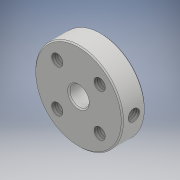
# Autodesk Inventor part: pololu-mounting-hub
Saved by Autodesk Inventor 2018 (Build 220112000, 112)
## iProperties
Created: 2017-11-16
Part Number: pololu-mounting-hub
Material: Generic
Document SubType Name: Modeling
Designer: leo2a
Density: 1 g/cm^3
Appearance: Default
Author: leo2a
Autodesk Inventor part; units mm, degrees
ref_plane "YZ Plane" through (0, 0, 0) normal (1, 0, 0) x (0, 1, 0)
ref_plane "XZ Plane" through (0, 0, 0) normal (0, 1, 0) x (-1, 0, 0)
ref_plane "XY Plane" through (0, 0, 0) normal (0, 0, 1) x (1, 0, 0)
sketch "Sketch1" plane through (0, 0, 0) normal (0, 1, 0) x (-1, 0, 0)
  circle A0 centre (0, 0) radius 9.525
  dimension "d0" = 19.05
  constraints: 1 centre point, 1 coincident
  measures "d0" diameter of A0
extrude "Extrusion1" add sketch "Sketch1" along normal blind 5
sketch "Sketch2" plane through (0, 5, 0) normal (0, 1, 0) x (1, 0, 0)
  line L0 (0, 0) -> (0, 6.5)
  point P0 (-6.5, 0)
  point P1 (0, -6.5)
  point P2 (6.5, 0)
  dimension "d3" = 6.5
  dimension "d6" = 360
  constraints: 2 end point, 1 coincident, 1 vertical, 5 other
  measures "d3" distance of L0.start L0.end
hole "Hole1" at (0, 5, -6.5) at (0, 5, 6.5) at (-6.5, 5, 0) at (6.5, 5, 0) direction (0, -1, 0) diameter 2.459 end through all thread size "M3x0.5" class "6H" standard "ISO Metric profile"
sketch "Sketch3" plane through (0, 5, 0) normal (0, 1, 0) x (1, 0, 0)
  circle A0 centre (0, 0) radius 2.1
  dimension "d15" = 4.2
  constraints: 1 centre point, 1 coincident
  measures "d15" diameter of A0
extrude "Extrusion2" cut sketch "Sketch3" against normal through all
chamfer "Chamfer1" distance 0.25 angle 45 4 edges at (-2.1, 5, 0) (9.525, 5, 0) (9.525, 0, 0) (-2.1, 0, 0)
move or copy body "Move Body1" bodies to move or copy 1 copy no rotation origin (0, 0, 0) rotation axis (0, 1, 0) rotation angle 45
sketch "Sketch4" plane through (0, 0, 0) normal (1, 0, 0) x (0, 1, 0)
  line L0 (0, 0) -> (2.5, 0)
  dimension "d22" = 2.5
  constraints: 2 end point, 1 coincident, 1 horizontal
  measures "d22" distance of L0.start L0.end
hole "Hole2" at (0, 2.5, 0) direction (1, 0, 0) diameter 2.459 end through all thread size "M3x0.5" class "6H" standard "ISO Metric profile"
body "Solid1"
